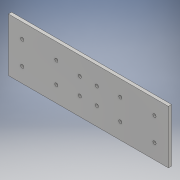
# Autodesk Inventor part: Góra
Saved by Autodesk Inventor 2017 (Build 210142000, 142)
## iProperties
Created: 2018-08-13
Part Number: Góra
Material: Aluminium 6061
Document SubType Name: Modeling
Designer: Wojciech
Density: 2.7 g/cm^3
Appearance: Aluminium — ciemne
Mass: 60.0629 g
Surface Area: 163.696 cm^2
Volume: 22.2455 cm^3
Author: Wojciech
Autodesk Inventor part; units mm, degrees
ref_plane "YZ Plane" through (0, 0, 0) normal (1, 0, 0) x (0, 1, 0)
ref_plane "XZ Plane" through (0, 0, 0) normal (0, 1, 0) x (-1, 0, 0)
ref_plane "XY Plane" through (0, 0, 0) normal (0, 0, 1) x (1, 0, 0)
sketch "Szkic1" plane through (0, 0, 0) normal (0, 1, 0) x (-1, 0, 0)
  line L0 (75, 25) -> (-75, 25)
  line L1 (-75, 25) -> (-75, -25)
  line L2 (-75, -25) -> (75, -25)
  line L3 (75, -25) -> (75, 25)
  line L4 (75, 25) -> (-75, -25) construction
  line L5 (-75, 25) -> (75, -25) construction
  point P0 (0, 0)
  dimension "d0" = 150
  dimension "d1" = 50
  constraints: 12 end point, 2 midpoint, 2 parallel, 1 horizontal, 1 perpendicular
  measures "d0" distance of L2.end L1.end
  measures "d1" distance of L1.end L0.end
extrude "Wyciągnięcie proste1" add sketch "Szkic1" along normal blind 3
sketch "Szkic3" plane through (0, 3, 0) normal (0, 1, 0) x (1, 0, 0)
  line L0 (75, 25) -> (-75, 25) projected
  line L1 (0, 25) -> (0, -25) construction
  line L2 (-75, -25) -> (75, -25) projected
  line L3 (-75, 25) -> (-75, -25) projected
  line L4 (-75, 0) -> (75, 0) construction
  line L5 (75, -25) -> (75, 25) projected
  point P0 (0, 0)
  point P1 (-30, 10)
  point P2 (30, 10)
  point P3 (-30, -10)
  point P4 (30, -10)
  dimension "d16" = 15
  dimension "d43" = 60
  constraints: 4 end point, 4 midpoint, 3 symmetric about line
  measures "d16" distance from line of L0 point (-30, 10)
  measures "d43" distance of point (-30, 10) point (30, 10)
hole "Otwór2" at (-30, 3, -10) at (30, 3, -10) at (-30, 3, 10) at (30, 3, 10) direction (0, -1, 0) diameter 3 depth 8 tip angle 118
sketch "Szkic4" plane through (0, 3, 0) normal (0, 1, 0) x (1, 0, 0)
  line L0 (75, -25) -> (75, 25) projected
  line L1 (-75, 25) -> (-75, -25) projected
  line L2 (-75, 0) -> (75, 0) construction
  line L3 (75, 25) -> (-75, 25) projected
  line L4 (0, 25) -> (0, -25) construction
  point P0 (0, 0)
  point P1 (62, 11)
  point P2 (62, -11)
  point P3 (-62, 11)
  point P4 (-62, -11)
  dimension "d24" = 13
  dimension "d25" = 11
  constraints: 4 end point, 3 midpoint, 3 symmetric about line, 1 vertical
  measures "d24" distance from line of L0 point (62, 11)
  measures "d25" distance from line of L2 point (62, 11)
hole "Otwór3" at (62, 3, -11) at (62, 3, 11) at (-62, 3, -11) at (-62, 3, 11) direction (0, -1, 0) diameter 3 depth 8 tip angle 118
sketch "Szkic5" plane through (0, 3, 0) normal (0, 1, 0) x (1, 0, 0)
  line L0 (-8, -8) -> (8, -8)
  line L1 (8, -8) -> (8, 8)
  line L2 (8, 8) -> (-8, 8)
  line L3 (-8, 8) -> (-8, -8)
  line L4 (-8, -8) -> (8, 8) construction
  line L5 (8, -8) -> (-8, 8) construction
  point P0 (0, 0)
  dimension "d33" = 16
  dimension "d34" = 16
  constraints: 12 end point, 4 coincident, 2 midpoint, 2 parallel, 1 horizontal, 1 perpendicular
  measures "d33" distance of L2.end L1.end
  measures "d34" distance of L1.end L0.end
hole "Otwór4" at (-8, 3, -8) at (8, 3, -8) at (8, 3, 8) at (-8, 3, 8) direction (0, -1, 0) diameter 3 depth 8 tip angle 118
